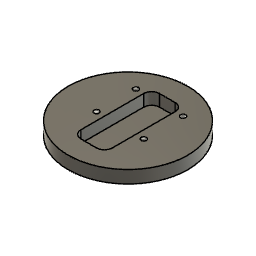
cryo bottom interface v2 (Autodesk Fusion 360 design; units mm, degrees)
Autodesk Fusion 360 part; units mm, degrees
sketch "Sketch1" plane through (0, 0, 0) normal (0, 1, 0) x (1, 0, 0)
  circle A0 centre (0, 0) radius 38
  line L0 (-10, 25) -> (10, 25)
  line L1 (10, 25) -> (10, -25)
  line L2 (10, -25) -> (-10, -25)
  line L3 (-10, -25) -> (-10, 25)
  line L4 (1.75, 0) -> (22.5, 0) construction
  line L5 (0, -1.75) -> (0, -22.5) construction
  dimension "d1" = 76
  dimension "d2" = 20
  dimension "d3" = 50
  constraint coincident A0.centre origin
  constraint horizontal L0
  constraint vertical L1
  constraint horizontal L2
  constraint vertical L3
  constraint symmetric L1 L3 L5
  constraint symmetric L0 L2 L4
  measures "d1" diameter of A0
  measures "d2" distance of L1.end L2.end
  measures "d3" distance of L0.end L1.end
extrude "Extrude1" add sketch "Sketch1" along normal blind 8
extrude "Extrude2" add sketch "Sketch1" along normal blind 0.5 contours L0 L1 L2 L3
sketch "Sketch2" plane through (0, 8, 0) normal (0, 1, 0) x (-1, 0, 0)
  line L0 (-10, 25) -> (10, 25)
  line L1 (10, 25) -> (10, -25)
  line L2 (10, -25) -> (-10, -25)
  line L3 (-10, -25) -> (-10, 25)
  circle A0 centre (0, 0) radius 38
  line L4 (0, 1.75) -> (0, 22.5)
  line L5 (-1.75, 0) -> (-22.5, 0)
  point P0 (15, -20)
  point P1 (15, 5)
  point P2 (-15, -20)
  point P3 (-15, 5)
  dimension "d10" = 30
  dimension "d11" = 25
  dimension "d12" = 20
  constraint horizontal P1 P3
  constraint horizontal P0 P2
  constraint vertical P0 P1
  constraint vertical P2 P3
  constraint symmetric P1 P3 L4
  measures "d10" distance of P0 P2
  measures "d11" distance of P0 P1
  measures "d12" distance of P2 L5
hole "Hole1" at (-15, 8, -20) at (-15, 8, 5) at (15, 8, -20) at (15, 8, 5) direction (0, -1, 0) diameter 3.332 depth 5 tip angle 118
thread "Thread1" "ISO Metric profile 4.0 M4x0.7 6H" thread offset 0 thread depth 10
fillet "Fillet1" radius 5 4 edges at (-10, 4.25, 25) (-10, 4.25, -25) (10, 4.25, 25) (10, 4.25, -25)
equation "d1 = ( 38 * 2 ) * 1 mm"
